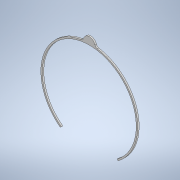
# Autodesk Inventor part: 69. Пружина синхронизатора
Saved by Autodesk Inventor 2021 (Build 250183000, 183)
## iProperties
Created: 2021-03-22
Part Number: 69. Пружина синхронизатора
Material: Типовые
Document SubType Name: Modeling
Designer: Данил
Density: 1 g/cm^3
Appearance: По умолчанию
Author: Данил
Autodesk Inventor part; units mm, degrees
ref_plane "YZ Plane" through (0, 0, 0) normal (1, 0, 0) x (0, 1, 0)
ref_plane "XZ Plane" through (0, 0, 0) normal (0, 1, 0) x (-1, 0, 0)
ref_plane "XY Plane" through (0, 0, 0) normal (0, 0, 1) x (1, 0, 0)
sketch "Эскиз1" plane through (0, 0, 0) normal (0, 0, 1) x (1, 0, 0)
  circle A0 centre (0, 0) radius 33
  circle A1 centre (0, 0) radius 32
  arc A2 (-5.4738, 32.5429) -> (-3.8704, 34.0101) centre (-5.8055, 34.5152) ccw
  arc A3 (3.8704, 34.0101) -> (-3.8704, 34.0101) centre (0, 33) ccw
  arc A4 (3.8704, 34.0101) -> (5.4738, 32.5429) centre (5.8055, 34.5152) ccw
  line L0 (-19, -25.7488) -> (19, -25.7488) construction
  line L1 (-19, -25.7488) -> (-19.8409, -26.3693)
  line L2 (19, -25.7488) -> (19.5938, -26.5534)
  arc A5 (-5.3079, 31.5567) -> (-2.9028, 33.7576) centre (-5.8055, 34.5152) ccw
  arc A6 (2.9028, 33.7576) -> (-2.9028, 33.7576) centre (0, 33) ccw
  arc A7 (2.9028, 33.7576) -> (5.3079, 31.5567) centre (5.8055, 34.5152) ccw
  dimension "d0" = 66
  dimension "d1" = 64
  dimension "d2" = 4
  dimension "d4" = 2
  dimension "d5" = 38
  constraints: 19 point on circle, 8 centre point, 6 end point, 5 tangent, 2 coincident, 1 equal radius, 1 horizontal, 1 horizontal alignment, 1 line through centre, 1 perpendicular, 2 other
  measures "d0" diameter of A0
  measures "d1" diameter of A1
  measures "d2" radius of A3
  measures "d4" radius of A4
  measures "d5" distance of L0.start L0.end
extrude "Выдавливание1" add sketch "Эскиз1" along normal mid plane 1 contours A0 L2 A1 A7 | A0 A7 A6 A5 A2 A3 A4 | A7 A1 A5 A0 | A0 A5 A6 A7 | A0 A5 A1 L1
